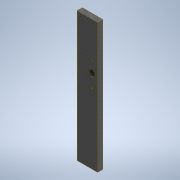
# Autodesk Inventor part: Placa4 Torre Tracera
Saved by Autodesk Inventor 2022 (Build 260153000, 153)
## iProperties
Created: 2021-11-08
Part Number: Placa4 Torre Tracera
Material: CFRP
Document SubType Name: Modeling
Designer: Samuel Gómez
Density: 1.43 g/cm^3
Appearance: Metal 2400F
Author: Samuel Gómez
Autodesk Inventor part; units mm, degrees
ref_plane "YZ Plane" through (0, 0, 0) normal (1, 0, 0) x (0, 1, 0)
ref_plane "XZ Plane" through (0, 0, 0) normal (0, 1, 0) x (-1, 0, 0)
ref_plane "XY Plane" through (0, 0, 0) normal (0, 0, 1) x (1, 0, 0)
sketch "Boceto1" plane through (0, 0, 0) normal (0, 0, 1) x (1, 0, 0)
  line L0 (0, 0) -> (70, 0)
  line L1 (70, 0) -> (70, 300)
  line L2 (70, 300) -> (0, 300)
  line L3 (0, 300) -> (0, 0)
  dimension "d0" = 300
  dimension "d1" = 70
  constraints: 8 end point, 2 parallel, 1 horizontal, 1 perpendicular
  measures "d0" distance of L2.end L0.start
  measures "d1" distance of L0.start L0.end
extrude "Extrusión1" add sketch "Boceto1" along normal blind 18
sketch "Boceto2" plane through (0, 0, 18) normal (0, 0, 1) x (1, 0, 0)
  circle A0 centre (50, 280) radius 11
  line L0 (70, 300) -> (0, 300) projected
  line L1 (70, 0) -> (70, 300) projected
  line L2 (50, 280) -> (50, 258) construction
  circle A1 centre (50, 258) radius 1.5
  line L3 (50, 280) -> (28, 280) construction
  circle A2 centre (28, 280) radius 1.5
  point P0 (0, 0)
  dimension "d4" = 22
  dimension "d6" = 20
  dimension "d7" = 3
  dimension "d8" = 22
  dimension "d9" = 22
  dimension "d10" = 3
  dimension "d11" = 20
  constraints: 4 end point, 3 centre point, 2 coincident, 1 horizontal, 1 vertical
  measures "d4" diameter of A0
  measures "d6" distance from line of L1 L2.start
  measures "d7" diameter of A1
  measures "d8" distance of L2.start L2.end
  measures "d9" distance of L2.start L3.end
  measures "d10" diameter of A2
  measures "d11" distance from line of L0 L2.start
extrude "Extrusión2" cut sketch "Boceto2" against normal blind 18
sketch "Boceto3" plane through (0, 0, 18) normal (0, 0, 1) x (1, 0, 0)
  line L0 (70, 300) -> (0, 300) projected
  line L1 (0, 300) -> (70, 300)
  line L2 (70, 300) -> (70, 440)
  line L3 (70, 440) -> (0, 440)
  line L4 (0, 440) -> (0, 300)
  circle A0 centre (50, 258) radius 1.5 projected
  circle A1 centre (50, 280) radius 11 projected
  line L5 (50, 258) -> (50, 280) construction
  circle A2 centre (28, 280) radius 1.5 projected
  line L6 (50, 280) -> (28, 280) construction
  point P0 (0, 0)
  dimension "d14" = 70
  dimension "d15" = 140
  constraints: 12 end point, 2 parallel, 2 perpendicular, 1 horizontal, 1 vertical
  measures "d14" distance of L2.end L3.end
  measures "d15" distance of L1.end L2.end
extrude "Extrusión3" add sketch "Boceto3" against normal up to surface (18 mm away) contours L0 L4 L3 L2
sketch "Boceto4" plane through (0, 0, 18) normal (0, 0, 1) x (1, 0, 0)
  circle A0 centre (50, 258) radius 1.5 projected
  line L0 (50, 258) -> (50, 302) construction
  circle A1 centre (28, 280) radius 1.5 projected
  line L1 (28, 280) -> (50, 280) construction
  circle A2 centre (50, 302) radius 1.5
  point P0 (0, 0)
  dimension "d19" = 22
  dimension "d20" = 3
  constraints: 4 end point, 1 centre point, 1 coincident, 1 midpoint, 1 perpendicular, 1 vertical
  measures "d19" distance from line of L0.end L1
  measures "d20" diameter of A2
extrude "Extrusión4" cut sketch "Boceto4" against normal blind 18 contours A2
sketch "Boceto5" plane through (0, 0, 18) normal (0, 0, 1) x (1, 0, 0)
  circle A0 centre (50, 240) radius 4
  circle A1 centre (50, 280) radius 11 projected
  circle A2 centre (50, 280) radius 11 projected
  line L0 (50, 280) -> (50, 193.7834) construction
  circle A3 centre (50, 320) radius 4
  line L1 (50, 320) -> (50, 280) construction
  point P0 (0, 0)
  dimension "d23" = 8
  dimension "d24" = 40
  dimension "d25" = 8
  dimension "d26" = 40
  constraints: 4 end point, 2 centre point, 2 vertical, 1 point on line
  measures "d23" diameter of A0
  measures "d24" distance of A0.centre A1.centre
  measures "d25" diameter of A3
  measures "d26" distance of L1.start L0.start
extrude "Extrusión5" cut sketch "Boceto5" against normal blind 18 contours A0 | A3
sketch "Boceto6" plane through (0, 0, 18) normal (0, 0, 1) x (1, 0, 0)
  circle A0 centre (50, 302) radius 1.5 projected
  circle A1 centre (50, 302) radius 1.5
  circle A2 centre (28, 280) radius 1.5 projected
  circle A3 centre (28, 280) radius 1.5
  circle A4 centre (50, 258) radius 1.5 projected
  circle A5 centre (50, 258) radius 1.5
  point P0 (0, 0)
  constraints: 3 centre point, 3 coincident
extrude "Extrusión6" add sketch "Boceto6" against normal up to surface (18 mm away)
